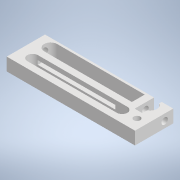
# Autodesk Inventor part: bottom slot
Saved by Autodesk Inventor 2020 (Build 240168000, 168)
## iProperties
Created: 2019-11-08
Part Number: bottom slot
Material: Generic
Document SubType Name: Modeling
Designer: Hymowitz
Density: 1 g/cm^3
Appearance: Default
Author: Hymowitz
Autodesk Inventor part; units mm, degrees
ref_plane "YZ Plane" through (0, 0, 0) normal (1, 0, 0) x (0, 1, 0)
ref_plane "XZ Plane" through (0, 0, 0) normal (0, 1, 0) x (-1, 0, 0)
ref_plane "XY Plane" through (0, 0, 0) normal (0, 0, 1) x (1, 0, 0)
sketch "Sketch1" plane through (0, 0, 0) normal (0, 1, 0) x (-1, 0, 0)
  line L0 (31.75, -3.048) -> (-31.75, -3.048)
  line L1 (-31.75, -3.048) -> (-31.75, 0)
  line L2 (-31.75, 0) -> (31.75, 0)
  line L3 (31.75, 0) -> (31.75, -3.048)
  line L4 (-31.75, 0) -> (31.75, 0)
  line L5 (31.75, 0) -> (31.75, 16.5722)
  line L6 (31.75, 16.5722) -> (-31.75, 16.5722)
  line L7 (-31.75, 16.5722) -> (-31.75, 0)
  line L8 (24.7167, 10.8097) -> (-19.6375, 10.8097) construction
  line L9 (24.7167, 13.3972) -> (-19.6375, 13.3972)
  line L10 (-19.6375, 8.2222) -> (24.7167, 8.2222)
  arc A0 (24.7167, 8.2222) -> (24.7167, 13.3972) centre (24.7167, 10.8097) ccw
  arc A1 (-19.6375, 13.3972) -> (-19.6375, 8.2222) centre (-19.6375, 10.8097) ccw
  line L11 (24.7167, 4.2534) -> (-24.7167, 4.2534) construction
  line L12 (24.7167, 6.6347) -> (-24.7167, 6.6347)
  line L13 (-24.7167, 1.8722) -> (24.7167, 1.8722)
  arc A2 (24.7167, 1.8722) -> (24.7167, 6.6347) centre (24.7167, 4.2534) ccw
  arc A3 (-24.7167, 6.6347) -> (-24.7167, 1.8722) centre (-24.7167, 4.2534) ccw
  line L14 (0, 0) -> (0, 22.7513) construction
  circle A4 centre (-26.9875, 10.8097) radius 1.5875
  point P0 (0, 4.2534)
  dimension "d5" = 49.4334
  dimension "d6" = 5.175
  dimension "d7" = 4.7625
  dimension "d8" = 4.2534
  dimension "d23" = 7.0333
  dimension "d24" = 3.175
  dimension "d25" = 3.175
  dimension "d26" = 3.175
  dimension "d27" = 1.5875
  dimension "d28" = 3.175
  constraints: 34 end point, 8 point on circle, 8 tangent, 5 centre point, 5 horizontal, 4 parallel, 3 vertical, 2 point on line, 1 collinear, 1 midpoint, 1 perpendicular, 4 other
  measures "d5" distance of L11.start L11.end
  measures "d6" distance between parallel lines of L9 L10
  measures "d7" distance between parallel lines of L13 L12
  measures "d8" distance between parallel lines of L2 L11
  measures "d23" distance from line of L5 L8.start
  measures "d24" diameter of A4
  measures "d25" distance edge to line of A4 L7
  measures "d27" distance between parallel lines of L12 L10
  measures "d28" distance between parallel lines of L6 L9
extrude "Extrusion1" add sketch "Sketch1" along normal mid plane 6.35 contours L2 L7 L6 L5
sketch "Sketch3" plane through (0, 3.175, 0) normal (0, 1, 0) x (1, 0, 0)
  arc A0 (24.7167, -6.6347) -> (24.7167, -1.8722) centre (24.7167, -4.2534) ccw projected
  line L0 (24.7167, -4.2534) -> (4.7773, -4.2534) construction
  line L1 (26.045, -9.5942) -> (22.235, -9.5942)
  line L2 (22.235, -9.5942) -> (22.235, 1.0874)
  line L3 (22.235, 1.0874) -> (26.045, 1.0874)
  line L4 (26.045, 1.0874) -> (26.045, -9.5942)
  line L5 (26.045, -9.5942) -> (22.235, 1.0874) construction
  line L6 (22.235, -9.5942) -> (26.045, 1.0874) construction
  point P0 (0, 0)
  point P1 (24.14, -4.2534)
  dimension "d14" = 10.6816
  dimension "d15" = 3.81
  constraints: 14 end point, 2 horizontal, 2 midpoint, 2 parallel, 1 perpendicular, 1 point on line
  measures "d14" distance of L3.end L1.start
  measures "d15" distance of L1.start L1.end
extrude "Extrusion3" cut sketch "Sketch3" against normal through all contours L4 L1 L2 L3
sketch "Sketch4" plane through (0, 3.175, 0) normal (0, 1, 0) x (1, 0, 0)
  line L0 (22.235, -6.6347) -> (-24.7167, -6.6347) projected
  line L1 (22.235, -1.8722) -> (-24.7167, -1.8722) projected
  line L2 (22.235, -6.6347) -> (18.6822, -6.6347)
  line L3 (18.6822, -6.6347) -> (18.6822, -1.8722)
  line L4 (18.6822, -1.8722) -> (22.235, -1.8722)
  line L5 (22.235, -1.8722) -> (22.235, -6.6347)
  point P0 (0, 0)
  point P1 (22.235, -1.8722)
  point P2 (18.6822, -6.6347)
  constraints: 8 end point, 2 parallel, 1 horizontal, 1 perpendicular, 1 point on line
extrude "Extrusion4" add sketch "Sketch4" against normal up to surface (6.35 mm away)
sketch "Sketch2" plane through (31.75, -3.175, 0) normal (1, 0, 0) x (0, 0, -1)
  line L0 (0, 3.175) -> (-16.5722, 3.175) construction
  line L1 (-16.5722, 6.35) -> (-16.5722, 0) construction
  line L2 (-6.6347, 0) -> (-6.6347, 6.35) construction
  line L3 (-1.8722, 6.35) -> (-1.8722, 0) construction
  circle A0 centre (-4.2534, 3.175) radius 1.5875
  line L4 (-6.6347, 0) -> (-6.6347, 6.35) construction
  line L5 (-6.6347, -1.3931) -> (-4.2534, -1.3931) construction
  line L6 (-1.8722, 0) -> (-1.8722, 6.35) construction
  line L7 (-1.8722, -1.3931) -> (-4.2534, -1.3931) construction
  line L8 (-4.2534, -1.3931) -> (-4.2534, 6.8506) construction
  line L9 (-6.6347, 6.35) -> (-6.6347, 0) projected
  line L10 (-1.8722, 0) -> (-1.8722, 6.35) projected
  point P0 (-7.4284, 6.35)
  point P1 (-7.4284, 0)
  dimension "d9" = 3.175
  constraints: 8 end point, 4 point on line, 1 centre point, 1 collinear, 1 horizontal, 1 midpoint, 1 perpendicular, 1 vertical, 2 other
  measures "d9" diameter of A0
extrude "Extrusion2" cut sketch "Sketch2" against normal through all
sketch "Sketch5" plane through (-24.7167, 3.175, 8.2222) normal (0, 0, 1) x (1, 0, 0)
  line L0 (24.7167, -3.175) -> (0, -3.175) construction
  line L1 (0, -6.35) -> (0, 0) construction
  line L2 (38.3736, -4.175) -> (0, -4.175)
  line L3 (0, -4.175) -> (0, -2.175)
  line L4 (0, -2.175) -> (38.3736, -2.175)
  line L5 (38.3736, -2.175) -> (38.3736, -4.175)
  line L6 (38.3736, -4.175) -> (0, -2.175) construction
  line L7 (0, -4.175) -> (38.3736, -2.175) construction
  line L8 (0, -6.35) -> (43.3989, -6.35) projected
  line L9 (43.3989, 0) -> (0, 0) projected
  point P0 (19.1868, -3.175)
  dimension "d18" = 2
  dimension "d21" = 2.175
  dimension "d22" = 2.175
  constraints: 14 end point, 3 midpoint, 2 parallel, 2 point on line, 1 horizontal, 1 perpendicular
  measures "d18" distance between parallel lines of L4 L2
  measures "d21" distance between parallel lines of L8 L2
  measures "d22" distance between parallel lines of L9 L4
extrude "Extrusion5" cut sketch "Sketch5" against normal up to next
body "Solid1"
